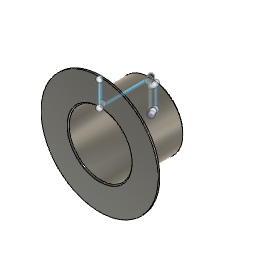
Kurbelgriff für Bürotisch ESB v14 (Autodesk Fusion 360 design; units mm, degrees)
Autodesk Fusion 360 part; units mm, degrees
ref_plane "Arbeitsebene11" through (0, 0, 3) normal (0, 0, 1) x (1, 0, 0)
sketch "Skizze34" plane through (0, 0, 3) normal (0, 0, 1) x (1, 0, 0)
  line L0 (0, 0) -> (0, 3) construction
  line L1 (0, 3.0015, 0.5015) -> (0, 3.0038, 1.3014)
  line L2 (0, 3.5038, 1.8) -> (0, 7.6485, 1.8)
  line L3 (0, 0, 0) -> (0, 0, 44) construction
  line L4 (0, 3.5069, 44) -> (0, 8.9068, 44)
  line L5 (0, 3.0069, 43.4932) -> (0, 3.0178, 42.6933)
  line L6 (0, 3.5178, 42.2002) -> (0, 7.1311, 42.2002)
  line L7 (0, 7.631, 41.7067) -> (0, 8.1484, 2.3066)
  line L8 (0, 3.5015) -> (0, 7.9725)
  line L9 (0, 9.4067, 43.5068) -> (0, 9.9724, 2.0273)
  arc A0 through (0, 9.9724, 2.0273) (0, 9.3964, 0.5955) (0, 7.9725, 0)
  arc A1 through (0, 7.6485, 1.8) (0, 8.0043, 1.9488) (0, 8.1484, 2.3066)
  arc A2 through (0, 3.0038, 1.3014) (0, 3.1507, 1.6541) (0, 3.5038, 1.8)
  arc A3 through (0, 3.5015, 0) (0, 3.1474, 0.147) (0, 3.0015, 0.5015)
  arc A4 through (0, 3.5038, 1.8) (0, 3.1507, 1.6541) (0, 3.0038, 1.3014)
  arc A5 through (0, 3.5015, 0) (0, 3.1474, 0.147) (0, 3.0015, 0.5015)
  arc A6 through (0, 3.0178, 42.6933) (0, 3.1666, 42.3442) (0, 3.5178, 42.2002)
  arc A7 through (0, 3.5069, 44) (0, 3.1509, 43.8511) (0, 3.0069, 43.4932)
  arc A8 through (0, 7.631, 41.7067) (0, 7.4823, 42.056) (0, 7.1311, 42.2002)
  arc A9 through (0, 9.4067, 43.5068) (0, 9.2579, 43.856) (0, 8.9068, 44)
  dimension "d120" = 3
  dimension "d123" = 44
  dimension "d131" = 2
  dimension "d133" = 0.5
  dimension "d134" = 0.5
  dimension "d135" = 0.5
  dimension "d136" = 0.5
  dimension "d137" = 0.5
  dimension "d138" = 0.5
  dimension "d139" = 0.5
  dimension "d140" = 0.5
  constraint coincident L0.start origin
  constraint vertical L0
  constraint coincident L0.end L8
  measures "d120" distance of L0.start L0.end
  measures "d123" distance of L0.start origin
revolve "Drehen2" add sketch "Skizze34" angle 360 about axis through (0, 0, 3) along (0, 0, 1) contours L1 L2 L4 L5 L6 L7 L8 L9 A0 A1 A2 A3 A4 A5 A6 A7 A8 A9 in plane through (0, 0, 3) normal (1, 0, 0) makes body 1
sketch "Skizze67" plane through (0, 0, 0) normal (1, 0, 0) x (0, 1, 0)
  line L0 (0, 0) -> (-1.5, 0)
  line L1 (-1.5, 0) -> (1.85, 0) construction
  line L2 (-2.98, 2.9) -> (-3.1672, 2.9)
  line L3 (-2.98, 2.9) -> (-2.98, 47.4)
  line L4 (-2.98, 47.4) -> (-2.38, 47.4)
  line L5 (-2.38, 47.4) -> (-2.38, 48.9)
  line L6 (-2.38, 48.9) -> (-2.98, 48.9)
  line L7 (0, 0) -> (0, 59.4)
  line L8 (-1.5, 0) -> (-3.1672, 2.9)
  line L9 (-2.98, 48.9) -> (-2.98, 56.734)
  line L10 (-4.98, 58.734) -> (-93.96, 58.734)
  line L11 (-2, 61.4) -> (-90.98, 61.4)
  line L12 (-92.98, 63.4) -> (-92.98, 109.38)
  line L13 (-95.96, 60.734) -> (-95.96, 109.378)
  line L14 (-92.98, 109.38) -> (-95.96, 109.378)
  arc A0 (0, 59.4) -> (-2, 61.4) centre (-2, 59.4) ccw
  arc A1 (-2.98, 56.734) -> (-4.98, 58.734) centre (-4.98, 56.734) ccw
  arc A2 (-95.96, 60.734) -> (-93.96, 58.734) centre (-93.96, 60.734) ccw
  arc A3 (-92.98, 63.4) -> (-90.98, 61.4) centre (-90.98, 63.4) ccw
  point P0 (0, 61.4)
  point P1 (-2.98, 58.734)
  point P2 (-95.96, 58.734)
  point P3 (-92.98, 61.4)
  dimension "d213" = 1.5
  dimension "d217" = 44.5
  dimension "d218" = 0.6
  dimension "d219" = 1.5
  dimension "d220" = 0.6
  dimension "d221" = 61.4
  dimension "d222" = 9.834
  dimension "d225" = 92.98
  dimension "d228" = 92.98
  dimension "d230" = 50.644
  dimension "d231" = 2
  constraint coincident L0.start L7.start
  constraint horizontal L0
  constraint horizontal L1
  constraint perpendicular L2 L3
  constraint perpendicular L3 L4
  constraint perpendicular L4 L5
  constraint perpendicular L5 L6
  constraint perpendicular L6 L9
  constraint perpendicular L9 L10
  constraint perpendicular L7 L11
  constraint perpendicular L10 L12
  constraint perpendicular L10 L13
  constraint coincident P0 L7
  constraint coincident P0 L11
  constraint tangent L7 A0
  constraint tangent L11 A0
  constraint coincident P1 L9
  constraint coincident P1 L10
  constraint tangent L9 A1
  constraint tangent L10 A1
  constraint equal A0 A1
  constraint coincident P2 L10
  constraint coincident P2 L13
  constraint tangent L10 A2
  constraint tangent L13 A2
  constraint equal A0 A2
  constraint coincident P3 L11
  constraint coincident P3 L12
  constraint tangent L11 A3
  constraint tangent L12 A3
  constraint equal A0 A3
  measures "d213" distance of L0.start L0.end
  measures "d217" distance of L2.start L3.end
  measures "d218" distance of L3.end L4.end
  measures "d219" distance of L4.end L5.end
  measures "d220" distance of L5.end L6.end
  measures "d221" distance of L0.start P0
  measures "d222" distance of L6.end P1
  measures "d225" distance of P1 P2
  measures "d228" distance of P0 P3
  measures "d230" distance of P2 L13.end
  measures "d231" radius of A0
sketch "Skizze70" plane through (0, 0, 0) normal (1, 0, 0) x (0, 1, 0)
  line L0 (-95.9615, 58.8292) -> (-95.9615, 105.3792)
  dimension "d227" = 46.55
  constraint vertical L0
  measures "d227" distance of L0.start L0.end
revolve "Drehen6" add sketch "Skizze67" angle 360 about axis through (0, -1.5, 0) along (0, 1, 0) separate body makes body 2
named bodies: "Schwarzer Kunstoff Kurbelgriff (1)", "Aluminium Kurbel"
